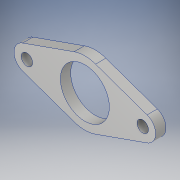
# Autodesk Inventor part: Axle Gear brace
Saved by Autodesk Inventor 2019.4 (Build 234330000, 330)
## iProperties
Created: 2020-01-13
Part Number: Axle Gear brace
Material: Aluminum 6061
Document SubType Name: Modeling
Designer: admin
Density: 2.7 g/cm^3
Appearance: Aluminum - Flat
Author: admin
Autodesk Inventor part; units mm, degrees
ref_plane "YZ Plane" through (0, 0, 0) normal (1, 0, 0) x (0, 1, 0)
ref_plane "XZ Plane" through (0, 0, 0) normal (0, 1, 0) x (-1, 0, 0)
ref_plane "XY Plane" through (0, 0, 0) normal (0, 0, 1) x (1, 0, 0)
sketch "Sketch1" plane through (0, 0, 0) normal (0, 0, 1) x (1, 0, 0)
  circle A0 centre (0, 0) radius 9.5
  arc A1 (-4.1667, 11.7851) -> (-4.1667, -11.7851) centre (0, 0) ccw construction
  circle A2 centre (22.5, 0) radius 2.2
  circle A3 centre (-22.5, 0) radius 2.2
  line L0 (-22.5, 0) -> (22.5, 0) construction
  arc A4 (-24.1667, -4.714) -> (-24.1667, 4.714) centre (-22.5, 0) ccw construction
  arc A5 (24.1667, 4.714) -> (24.1667, -4.714) centre (22.5, 0) ccw construction
  line L1 (24.1667, 4.714) -> (4.1667, 11.7851)
  line L2 (-24.1667, 4.714) -> (-4.1667, 11.7851)
  line L3 (-24.1667, -4.714) -> (-4.1667, -11.7851)
  line L4 (4.1667, -11.7851) -> (24.1667, -4.714)
  arc A6 (-24.1667, 4.714) -> (-24.1667, -4.714) centre (-22.5, 0) ccw
  arc A7 (4.1667, 11.7851) -> (-4.1667, 11.7851) centre (0, 0) ccw
  arc A8 (4.1667, -11.7851) -> (4.1667, 11.7851) centre (0, 0) ccw construction
  arc A9 (-4.1667, -11.7851) -> (4.1667, -11.7851) centre (0, 0) ccw
  arc A10 (24.1667, -4.714) -> (24.1667, 4.714) centre (22.5, 0) ccw
  dimension "d0" = 19
  dimension "d1" = 25
  dimension "d2" = 4.4
  dimension "d3" = 4.4
  dimension "d4" = 45
  dimension "d5" = 10
  dimension "d6" = 10
  constraints: 17 point on circle, 11 centre point, 10 end point, 9 tangent, 5 coincident, 2 parallel, 1 horizontal, 1 midpoint
  measures "d0" diameter of A0
  measures "d1" diameter of A1
  measures "d2" diameter of A2
  measures "d3" diameter of A3
  measures "d4" distance of L0.start L0.end
  measures "d5" diameter of A4
  measures "d6" diameter of A5
extrude "Extrusion1" add sketch "Sketch1" along normal blind 4
body "Solid1"
